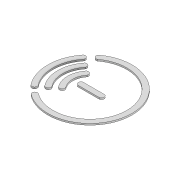
# Autodesk Inventor part: BordaLogo
Saved by Autodesk Inventor 2020.3 (Build 243373000, 373)
## iProperties
Created: 2021-08-24
Part Number: BordaLogo
Material: Generic
Document SubType Name: Modeling
Designer: Yusuf
Mass: 5.59154 g
Surface Area: 73.9053 cm^2
Volume: 5.59154 cm^3
Density: 1 g/cm^3
Appearance: Default
Author: Yusuf
Autodesk Inventor part; units mm, degrees
ref_plane "YZ Plane" through (0, 0, 0) normal (1, 0, 0) x (0, 1, 0)
ref_plane "XZ Plane" through (0, 0, 0) normal (0, 1, 0) x (-1, 0, 0)
ref_plane "XY Plane" through (0, 0, 0) normal (0, 0, 1) x (1, 0, 0)
sketch "Sketch1" plane through (0, 0, 0) normal (0, 1, 0) x (-1, 0, 0)
  circle A0 centre (0, 0) radius 53.85
  circle A1 centre (0, 0) radius 47.25
  circle A2 centre (0, 0) radius 41.25
  circle A3 centre (0, 0) radius 28.65
  circle A4 centre (0, 0) radius 22.05
  circle A5 centre (0, 0) radius 34.65
  line L0 (0, 53.85) -> (0, -53.85) construction
  line L1 (0, 0) -> (42.1434, -33.5224)
  line L2 (0, 0) -> (32.4077, -43.0065)
  arc A6 (36.9782, -29.4138) -> (42.1434, -33.5224) centre (40.0704, -30.8275) ccw
  line L3 (39.5608, -31.4681) -> (39.9924, -30.9256) construction
  arc A7 (27.1174, -21.5701) -> (32.2826, -25.6787) centre (30.2095, -22.9838) ccw
  arc A8 (17.2565, -13.7264) -> (22.4217, -17.835) centre (20.3487, -15.1402) ccw
  arc A9 (32.4077, -43.0065) -> (28.4358, -37.7355) centre (29.6124, -40.9809) ccw
  line L4 (0, 0) -> (42.1434, 33.5224)
  line L5 (0, 0) -> (32.4077, 43.0065)
  arc A10 (42.1434, 33.5224) -> (36.9782, 29.4138) centre (40.0704, 30.8275) ccw
  line L6 (39.5608, 31.4681) -> (39.9924, 30.9256) construction
  arc A11 (32.2826, 25.6787) -> (27.1174, 21.5701) centre (30.2095, 22.9838) ccw
  arc A12 (22.4217, 17.835) -> (17.2565, 13.7264) centre (20.3487, 15.1402) ccw
  arc A13 (28.4358, 37.7355) -> (32.4077, 43.0065) centre (29.6124, 40.9809) ccw
  line L7 (47.25, 0) -> (41.25, 0)
  line L8 (34.65, 0) -> (28.65, 0)
  line L9 (22.05, 0) -> (-53.85, 0)
  line L10 (53.6613, -53.4353) -> (53.6613, 53.4353)
  line L11 (0, 0) -> (88.3768, 0)
  line L12 (12.0694, -3.3) -> (-15.3926, -3.3)
  line L13 (12.0694, 3.3) -> (-15.3926, 3.3)
  line L14 (8.2219, -3.3) -> (8.2219, 3.3)
  arc A14 (12.0694, -3.3) -> (12.0694, 3.3) centre (11.4617, 0) ccw
  arc A15 (-15.3926, 3.3) -> (-15.3926, -3.3) centre (-14.7876, 0) ccw
  point P0 (53.6613, 0)
  point P1 (0, 53.4353)
  point P2 (8.2219, 0)
  point P3 (32.4077, 43.0065)
  point P4 (27.1174, 21.5701)
  point P5 (53.6613, 4.5036)
  point P6 (36.9782, 29.4138)
  point P7 (53.6613, -4.5036)
  dimension "d3" = 94.5
  dimension "width" = 6.6
  dimension "d7" = 6.6
  dimension "d8" = 6.6
  dimension "d11" = 6
  dimension "d13" = 6
  dimension "d31" = 3.4
  dimension "d59" = 6.6
  dimension "d60" = 3.3555
  dimension "d62" = 3.355
  constraints: 36 point on circle, 30 end point, 19 point on line, 16 centre point, 6 coincident, 6 horizontal, 3 perpendicular, 2 equal radius, 2 horizontal alignment, 2 midpoint, 1 vertical, 1 vertical alignment
  measures "d3" diameter of A1
  measures "width" radial gap between concentric circles of A1 A0
  measures "d7" radial gap between concentric circles of A4 A3
  measures "d8" radial gap between concentric circles of A5 A2
  measures "d11" radial gap between concentric circles of A2 A1
  measures "d13" radial gap between concentric circles of A3 A5
  measures "d31" radius of A6
  measures "d59" distance between parallel lines of L13 L12
  measures "d60" radius of A14
  measures "d62" radius of A15
extrude "Extrusion1" add sketch "Sketch1" along normal blind 2 contours A0 L10 L11 A1 L4 | L4 A10 | L5 A1 L9 A0 | A13 L5 | L9 A1 L2 A0 | L10 A0 L1 A1 L11 | A2 L11 A5 L4 | L4 A11 | L2 A9 | L1 A6 | A2 L1 A5 L11 | A7 L1 | A3 L11 A4 L4 | L4 A12 | A3 L1 A4 L11 | A8 L1 | L13 L14 L9 L4 | L4 L5 L13 | L5 L9 A15 L13 | A14 L12 L14 L9 | L9 L14 L13 A14 | L9 L14 L12 L1 | L1 L12 L2 | L2 L12 A15 L9
equation "\"d7\" = width"
equation "\"d8\" = width"
body "Solid1"
